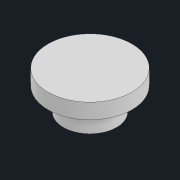
# Autodesk Inventor part: FijadorParaBloqueo
Saved by Autodesk Inventor 2021 (Build 250183000, 183)
## iProperties
Created: 2021-05-06
Part Number: FijadorParaBloqueo
Material: Generic
Document SubType Name: Modeling
Designer: GABRIEL LOL
Density: 1 g/cm^3
Appearance: Default
Author: GABRIEL LOL
Autodesk Inventor part; units mm, degrees
ref_plane "YZ Plane" through (0, 0, 0) normal (1, 0, 0) x (0, 1, 0)
ref_plane "XZ Plane" through (0, 0, 0) normal (0, 1, 0) x (-1, 0, 0)
ref_plane "XY Plane" through (0, 0, 0) normal (0, 0, 1) x (1, 0, 0)
sketch "Sketch1" plane through (0, 0, 0) normal (0, 0, 1) x (1, 0, 0)
  line L0 (0, 0) -> (1.5, 0)
  line L1 (1.5, 0) -> (1.5, 3)
  line L2 (1.5, 3) -> (5.5, 3)
  line L3 (5.5, 3) -> (5.5, 5)
  line L4 (5.5, 5) -> (0, 5)
  line L5 (0, 5) -> (0, 3)
  line L6 (0, 3) -> (1.5, 3)
  line L7 (1.5, 0) -> (3.5, 0)
  line L8 (3.5, 0) -> (3.5, 3)
  line L9 (0, -1) -> (0, 6) projected
  dimension "d0" = 1.5
  dimension "d1" = 3
  dimension "d2" = 4
  dimension "d3" = 2
  dimension "d4" = 2
  constraints: 18 end point, 4 perpendicular, 3 horizontal, 1 collinear, 1 midpoint, 1 point on line
  measures "d0" distance of L0.start L0.end
  measures "d1" distance of L0.end L1.end
  measures "d2" distance of L1.end L2.end
  measures "d3" distance of L2.end L3.end
  measures "d4" distance of L0.end L7.end
revolve "Revolution1" add sketch "Sketch1" angle 360 about axis through (0, -10, 0) along (0, 1, 0) contours L1 L2 L8 L7 | L5 L4 L3 L2 L6
thread "Thread1" size "M3x0.5" class "6H" standard "ISO Metric profile" full length
body "Solid1"
